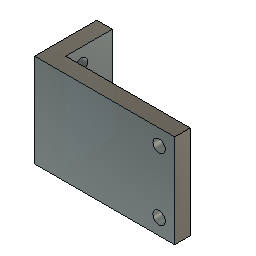
y-limit switch v2 (Autodesk Fusion 360 design; units mm, degrees)
Autodesk Fusion 360 part; units mm, degrees
sketch "Skizze1" plane through (0, 0, 0) normal (0, 0, 1) x (1, 0, 0)
  line L0 (0, 0) -> (20, 0)
  line L1 (20, 0) -> (20, 20)
  line L2 (20, 20) -> (0, 20)
  line L3 (0, 20) -> (0, 0)
  line L4 (0, 20) -> (0, 25)
  line L5 (0, 25) -> (25, 25)
  line L6 (25, 25) -> (25, 0)
  line L7 (20, 0) -> (25, 0)
  dimension "d1" = 20
  dimension "d2" = 20
  constraint horizontal L0
  constraint vertical L1
  constraint horizontal L2
  constraint vertical L3
  constraint coincident L0.start L3.end
  constraint perpendicular L2 L4
  constraint perpendicular L4 L5
  constraint perpendicular L5 L6
  constraint perpendicular L6 L7
  measures "d1" distance of L0.start L0.end
  measures "d2" distance of L0.start L2.end
extrude "Extrusion1" add sketch "Skizze1" along normal blind 30 contours L1 L2 L4 L5 L6 L7 makes body 1
sketch "Skizze2" plane through (0, 25, 0) normal (0, 1, 0) x (-1, 0, 0)
  line L0 (-25, 0) -> (0, 0)
  line L1 (0, 0) -> (0, 30)
  line L2 (0, 30) -> (-25, 30)
  line L3 (-25, 30) -> (-25, 0)
sketch "Skizze3" plane through (25, 0, 0) normal (1, 0, 0) x (0, 1, 0)
  line L0 (0, 0) -> (25, 0)
  line L1 (25, 0) -> (25, 30)
  line L2 (25, 30) -> (0, 30)
  line L3 (0, 30) -> (0, 0)
  line L4 (0, 30) -> (5, 30)
  line L5 (5, 30) -> (5, 0)
  line L6 (5, 0) -> (0, 0)
  line L7 (0, 0) -> (0, 30)
  constraint horizontal L4
  constraint vertical L5
  constraint horizontal L6
  constraint vertical L7
  constraint coincident L0 L5.end
  constraint coincident L2.end L3.start
extrude "Extrusion2" add sketch "Skizze3" along normal blind 40 contours L0 L2 L3 L4 L5 L6 L7 bodies 1
sketch "Skizze4" plane through (0, 0, 0) normal (0, -1, 0) x (1, 0, 0)
  line L0 (20, 0) -> (65, 0)
  line L1 (65, 0) -> (65, 30)
  line L2 (65, 30) -> (20, 30)
  line L3 (20, 30) -> (20, 0)
  circle A0 centre (60, 25) radius 2
  circle A1 centre (60, 5) radius 2
  dimension "d7" = 4
  dimension "d8" = 4
  measures "d7" diameter of A0
  measures "d8" diameter of A1
extrude "Extrusion3" cut sketch "Skizze4" against normal blind 12 contours A0 | A1 bodies 1
sketch "Skizze5" plane through (20, 0, 0) normal (-1, 0, 0) x (0, -1, 0)
  line L0 (-20, 0) -> (0, 0)
  line L1 (0, 0) -> (0, 30)
  line L2 (0, 30) -> (-20, 30)
  line L3 (-20, 30) -> (-20, 0)
  line L4 (0, 29) -> (-10, 29)
  circle A0 centre (-10, 25) radius 2
  circle A1 centre (-10, 5) radius 2
  dimension "d15" = 4
  dimension "d16" = 4
  constraint coincident L1 L4.start
  constraint perpendicular L3 L4
  measures "d15" diameter of A0
  measures "d16" diameter of A1
extrude "Extrusion4" cut sketch "Skizze5" against normal blind 7 contours A0 | A1 bodies 1
sketch "Skizze6" plane through (0, 20, 0) normal (0, -1, 0) x (1, 0, 0)
  line L0 (0, 0) -> (20, 0)
  line L1 (20, 0) -> (20, 30)
  line L2 (20, 30) -> (0, 30)
  line L3 (0, 30) -> (0, 0)
  circle A0 centre (10, 25) radius 2
  circle A1 centre (10, 5) radius 2
  line L4 (10, 20) -> (7, 20)
  line L5 (7, 20) -> (7, 10)
  line L6 (7, 10) -> (10, 10)
  line L7 (10, 10) -> (10, 20)
  line L8 (10, 20) -> (13, 20)
  line L9 (13, 20) -> (13, 10)
  line L10 (13, 10) -> (10, 10)
  line L11 (10, 10) -> (10, 20)
  dimension "d19" = 4
  dimension "d20" = 4
  constraint horizontal L4
  constraint vertical L5
  constraint horizontal L6
  constraint vertical L7
  constraint horizontal L8
  constraint vertical L9
  constraint horizontal L10
  constraint vertical L11
  measures "d19" diameter of A0
  measures "d20" diameter of A1
extrude "Extrusion5" add sketch "Skizze6" along normal blind 4 contours L4 L5 L6 L7 L11 | L7 L8 L9 L10 L11 bodies 1
sketch "Skizze7" plane through (0, 20, 0) normal (0, -1, 0) x (1, 0, 0)
  line L0 (13, 20) -> (13, 10)
  line L1 (13, 10) -> (7, 10)
  line L2 (7, 10) -> (7, 20)
  line L3 (7, 20) -> (13, 20)
  line L4 (0, 0) -> (20, 0)
  line L5 (20, 0) -> (20, 30)
  line L6 (20, 30) -> (0, 30)
  line L7 (0, 30) -> (0, 0)
  circle A0 centre (10, 25) radius 1.75
  circle A1 centre (10, 5) radius 1.75
  dimension "d23" = 3.5
  dimension "d24" = 3.5
  measures "d23" diameter of A0
  measures "d24" diameter of A1
extrude "Extrusion6" cut sketch "Skizze7" against normal blind 9 contours A0 | A1 bodies 1
sketch "Skizze9" plane through (0, 25, 0) normal (0, 1, 0) x (-1, 0, 0)
sketch "Skizze10" plane through (0, 25, 0) normal (0, 1, 0) x (-1, 0, 0)
extrude "Extrusion8" cut sketch "Skizze2" against normal blind 5 bodies 1 makes body 2 at (32.7327, 0, 11.9559)
extrude "Extrusion9" cut 1 faces at (7, 18.6667, 16.6667) along direction (1, 0, 0) blind 6 on bodies 1 bodies 1
sketch "Skizze11" plane through (20, 0, 0) normal (-1, 0, 0) x (0, -1, 0)
  circle A0 centre (-10, 25) radius 2
  circle A1 centre (-10, 5) radius 2
  line L0 (-20, 0) -> (0, 0)
  line L1 (0, 0) -> (0, 30)
  line L2 (0, 30) -> (-20, 30)
  line L3 (-20, 30) -> (-20, 0)
  line L4 (-10, 20) -> (-13, 20)
  line L5 (-13, 20) -> (-13, 10)
  line L6 (-13, 10) -> (-10, 10)
  line L7 (-10, 10) -> (-10, 20)
  line L8 (-10, 20) -> (-7, 20)
  line L9 (-7, 20) -> (-7, 10)
  line L10 (-7, 10) -> (-10, 10)
  line L11 (-10, 10) -> (-10, 20)
  constraint horizontal L4
  constraint vertical L5
  constraint horizontal L6
  constraint vertical L7
  constraint horizontal L8
  constraint vertical L9
  constraint horizontal L10
  constraint vertical L11
extrude "Extrusion10" add sketch "Skizze11" along normal blind 5 contours L4 L5 L6 L7 L11 | L7 L8 L9 L10 L11 bodies 1 2
sketch "Skizze12" plane through (25, 0, 0) normal (1, 0, 0) x (0, 1, 0)
  line L0 (20, 0) -> (20, 30)
  line L1 (20, 30) -> (5, 30)
  line L2 (5, 30) -> (5, 0)
  line L3 (5, 0) -> (20, 0)
  circle A0 centre (10, 5) radius 2
  circle A1 centre (10, 25) radius 2
sketch "Skizze13" plane through (0, 0, 0) normal (0, -1, 0) x (1, 0, 0)
  circle A0 centre (60, 25) radius 2
  circle A1 centre (60, 5) radius 2
  line L0 (20, 0) -> (65, 0)
  line L1 (65, 0) -> (65, 30)
  line L2 (65, 30) -> (20, 30)
  line L3 (20, 30) -> (20, 0)
